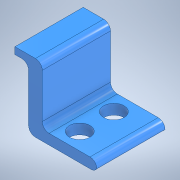
# Autodesk Inventor part: CableGuide
Saved by Autodesk Inventor 2021 (Build 250183000, 183)
## iProperties
Created: 2021-11-17
Part Number: CableGuide
Material: Generic
Document SubType Name: Modeling
Designer: Jorian Brusind
Density: 1 g/cm^3
Appearance: Cyan
Author: Jorian Brusind
Autodesk Inventor part; units mm, degrees
ref_plane "YZ Plane" through (0, 0, 0) normal (1, 0, 0) x (0, 1, 0)
ref_plane "XZ Plane" through (0, 0, 0) normal (0, 1, 0) x (-1, 0, 0)
ref_plane "XY Plane" through (0, 0, 0) normal (0, 0, 1) x (1, 0, 0)
sketch "Sketch1" plane through (0, 0, 0) normal (0, 1, 0) x (-1, 0, 0)
  line L0 (0, 0) -> (20, 0)
  line L1 (20, 0) -> (20, -20)
  line L2 (20, -20) -> (0, -20)
  line L3 (0, -20) -> (0, 0)
  dimension "d0" = 20
  dimension "d1" = 20
  constraints: 8 end point, 2 parallel, 1 horizontal, 1 perpendicular
  measures "d0" distance of L1.end L2.end
  measures "d1" distance of L0.end L1.end
extrude "Extrusion1" add sketch "Sketch1" along normal blind 3
sketch "Sketch2" plane through (0, 3, 0) normal (0, 1, 0) x (1, 0, 0)
  circle A0 centre (-10, 15) radius 3
  line L0 (0, 0) -> (0, 20) projected
  line L1 (0, 20) -> (-20, 20) projected
  circle A1 centre (-10, 5) radius 3
  dimension "d4" = 6
  dimension "d5" = 10
  dimension "d6" = 5
  dimension "d23" = 6
  dimension "d24" = 10
  dimension "d25" = 10
  constraints: 2 centre point
  measures "d4" diameter of A0
  measures "d5" distance from line of L0 A0.centre
  measures "d6" distance from line of L1 A0.centre
  measures "d23" diameter of A1
  measures "d24" distance of A0.centre A1.centre
  measures "d25" distance from line of L0 A1.centre
extrude "Extrusion2" cut sketch "Sketch2" against normal through all
sketch "Sketch3" plane through (0, 3, 0) normal (0, 1, 0) x (1, 0, 0)
  circle A0 centre (-10, 15) radius 3 projected
  circle A1 centre (-10, 15) radius 5
  line L0 (-10, 15) -> (-18, 15)
  line L1 (0, 20) -> (-20, 20) projected
  line L2 (-20, 0) -> (-16, 0)
  line L3 (-16, 0) -> (-16, 20)
  line L4 (-16, 20) -> (-20, 20)
  line L5 (-20, 20) -> (-20, 0)
  line L6 (0, 0) -> (0, 20) projected
  dimension "d9" = 10
  dimension "d10" = 8
  dimension "d11" = 4
  dimension "d26" = 20
  dimension "d27" = 20
  constraints: 10 end point, 2 horizontal, 2 parallel, 1 centre point, 1 coincident, 1 perpendicular, 1 point on line
  measures "d9" diameter of A1
  measures "d10" distance of L0.start L0.end
  measures "d11" distance of L4.end L3.end
  measures "d26" distance of L4.end L2.start
  measures "d27" distance between parallel lines of L6 L5
extrude "Extrusion3" add sketch "Sketch3" along normal blind 17 contours L3 L2 L5 L1
sketch "Sketch4" plane through (-20, 0, -20) normal (-1, 0, 0) x (0, 0, 1)
  line L0 (0, 0) -> (0, 20) projected
  line L1 (0, 20) -> (20, 20)
  line L2 (20, 20) -> (20, 18)
  line L3 (20, 18) -> (0, 18)
  line L4 (0, 18) -> (0, 20)
  point P0 (20, 0)
  dimension "d14" = 20
  dimension "d15" = 2
  constraints: 8 end point, 2 parallel, 1 horizontal, 1 perpendicular
  measures "d14" distance of L2.end L3.end
  measures "d15" distance of L1.end L2.end
extrude "Extrusion4" add sketch "Sketch4" along normal blind 4
fillet "Fillet1" radius 2 1 edges at (-16, 20, -10)
fillet "Fillet2" radius 2 1 edges at (-20, 18, -10)
fillet "Fillet3" radius 2 1 edges at (-20, 0, -10)
fillet "Fillet4" radius 2 1 edges at (-16, 3, -10)
fillet "Fillet5" radius 2 2 edges at (0, 3, -10) (0, 0, -10)
body "Solid1"
